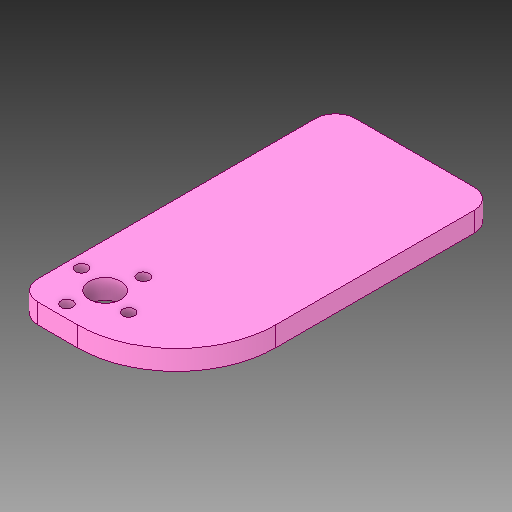
# Autodesk Inventor part: trappe
Saved by Autodesk Inventor 2017 (Build 210142000, 142)
## iProperties
Created: 2018-04-01
Part Number: trappe
Material: Generic
Document SubType Name: Modeling
Designer: franc
Density: 1 g/cm^3
Appearance: Default
Author: franc
Autodesk Inventor part; units mm, degrees
ref_plane "YZ Plane" through (0, 0, 0) normal (1, 0, 0) x (0, 1, 0)
ref_plane "XZ Plane" through (0, 0, 0) normal (0, 1, 0) x (-1, 0, 0)
ref_plane "XY Plane" through (0, 0, 0) normal (0, 0, 1) x (1, 0, 0)
sketch "Esquisse1" plane through (0, 0, 0) normal (0, 1, 0) x (-1, 0, 0)
  line L0 (16.0248, 37.2671) -> (-23.9752, 37.2671)
  line L1 (-23.9752, 37.2671) -> (-23.9752, -42.7329)
  line L2 (-23.9752, -42.7329) -> (16.0248, -42.7329)
  line L3 (16.0248, -42.7329) -> (16.0248, 37.2671)
  point P0 (0, 0)
  dimension "d0" = 80
  dimension "d1" = 40
  constraints: 8 end point, 2 parallel, 1 horizontal, 1 perpendicular
  measures "d0" distance of L2.end L0.start
  measures "d1" distance of L0.start L0.end
extrude "Extrusion1" add sketch "Esquisse1" along normal blind 5
sketch "Esquisse2" plane through (0, 0, 0) normal (0, -1, 0) x (1, 0, 0)
  point P0 (0, 0)
sketch "Esquisse3" plane through (0, 0, 0) normal (0, -1, 0) x (1, 0, 0)
  arc A0 (-2.5931, 17.1019) -> (-3.0796, 16.9864) centre (-3.1778, 18.4832) ccw projected
  circle A1 centre (-12.8087, 24.4201) radius 1.5 projected
  circle A2 centre (-6.8718, 34.0509) radius 1.5 projected
  circle A3 centre (2.759, 28.1141) radius 1.25 projected
  circle A4 centre (-5.0248, 26.2671) radius 4 projected
  circle A5 centre (-3.1778, 18.4832) radius 1.5
  circle A6 centre (2.759, 28.1141) radius 1.5
  point P0 (0, 0)
  dimension "d6" = 3
  constraints: 2 centre point, 2 coincident, 1 concentric
  measures "d6" diameter of A6
extrude "Extrusion2" cut sketch "Esquisse3" against normal through all contours A5 A0 | A1 | A2 | A3 | A4 | A6
fillet "Congé1" radius 25 1 edges at (23.9752, 2.5, 37.2671)
fillet "Congé2" radius 5 1 edges at (23.9752, 2.5, -42.7329)
fillet "Congé3" radius 5 1 edges at (-16.0248, 2.5, -42.7329)
fillet "Congé4" radius 5 1 edges at (-16.0248, 2.5, 37.2671)
